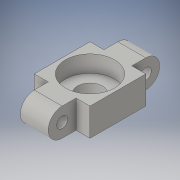
# Autodesk Inventor part: top_anchor_v3
Saved by Autodesk Inventor 2016 (Build 200138000, 138)
## iProperties
Created: 2016-02-24
Part Number: top_anchor_v3
Material: Generic
Document SubType Name: Modeling
Designer: Matt Ruffner
Density: 1 g/cm^3
Appearance: Default
Author: Matt Ruffner
Autodesk Inventor part; units mm, degrees
ref_plane "YZ Plane" through (0, 0, 0) normal (1, 0, 0) x (0, 1, 0)
ref_plane "XZ Plane" through (0, 0, 0) normal (0, 1, 0) x (-1, 0, 0)
ref_plane "XY Plane" through (0, 0, 0) normal (0, 0, 1) x (1, 0, 0)
sketch "Sketch1" plane through (0, 0, 0) normal (0, 1, 0) x (-1, 0, 0)
  line L0 (7.6182, 15.9234) -> (-17.7818, 15.9234)
  line L1 (-17.7818, 15.9234) -> (-17.7818, -34.8766)
  line L2 (-17.7818, -34.8766) -> (7.6182, -34.8766)
  line L3 (7.6182, -34.8766) -> (7.6182, 15.9234)
  line L4 (7.6182, 15.9234) -> (1.2682, 15.9234)
  line L5 (1.2682, 15.9234) -> (1.2682, 3.2234)
  line L6 (1.2682, 3.2234) -> (7.6182, 3.2234)
  line L7 (7.6182, 3.2234) -> (7.6182, 15.9234)
  line L8 (-17.7818, 15.9234) -> (-11.4318, 15.9234)
  line L9 (-11.4318, 15.9234) -> (-11.4318, 3.2234)
  line L10 (-11.4318, 3.2234) -> (-17.7818, 3.2234)
  line L11 (-17.7818, 3.2234) -> (-17.7818, 15.9234)
  line L12 (-17.7818, -34.8766) -> (-11.4318, -34.8766)
  line L13 (-11.4318, -34.8766) -> (-11.4318, -22.1766)
  line L14 (-11.4318, -22.1766) -> (-17.7818, -22.1766)
  line L15 (-17.7818, -22.1766) -> (-17.7818, -34.8766)
  line L16 (7.6182, -34.8766) -> (1.2682, -34.8766)
  line L17 (1.2682, -34.8766) -> (1.2682, -22.1766)
  line L18 (1.2682, -22.1766) -> (7.6182, -22.1766)
  line L19 (7.6182, -22.1766) -> (7.6182, -34.8766)
  circle A0 centre (-5.0818, -9.4766) radius 5.715
  point P0 (0, 0)
  dimension "d0" = 25.4
  dimension "d1" = 50.8
  dimension "d2" = 6.35
  dimension "d3" = 12.7
  dimension "d4" = 6.35
  dimension "d5" = 12.7
  dimension "d6" = 6.35
  dimension "d7" = 12.7
  dimension "d8" = 11.43
  constraints: 40 end point, 10 parallel, 5 horizontal, 5 perpendicular, 2 point on line, 1 centre point
  measures "d0" distance of L2.end L1.end
  measures "d1" distance of L1.end L0.end
  measures "d2" distance of L6.end L5.end
  measures "d3" distance of L5.end L4.end
  measures "d4" distance of L9.end L10.end
  measures "d5" distance of L13.end L12.end
  measures "d6" distance of L17.end L18.end
  measures "d7" distance of L16.end L17.end
  measures "d8" diameter of A0
extrude "Extrusion1" add sketch "Sketch1" along normal blind 12.7 contours L5 L6 L3 L18 L17 L2 L13 L14 L1 L10 L9 L0
sketch "Sketch2" plane through (11.4318, 0, 3.2234) normal (1, 0, 0) x (0, 0, -1)
  line L0 (-12.7, 0) -> (-12.7, 12.7) projected
  line L1 (-12.7, 12.7) -> (0, 12.7) projected
  line L2 (38.1, 12.7) -> (38.1, 0) projected
  circle A0 centre (-6.35, 6.35) radius 2.5083
  circle A1 centre (31.75, 6.35) radius 2.5082
  point P0 (3.2234, 0)
  dimension "d11" = 6.35
  dimension "d12" = 6.35
  dimension "d13" = 6.35
  dimension "d14" = 5.0165
  dimension "d15" = 5.0165
  constraints: 2 centre point, 2 coincident
  measures "d11" distance from line of L0 point (-6.35, 6.35)
  measures "d12" distance from line of point (-6.35, 6.35) L1
  measures "d13" distance from line of L2 point (31.75, 6.35)
  measures "d14" diameter of A0
  measures "d15" diameter of A1
extrude "Extrusion2" cut sketch "Sketch2" against normal through all
sketch "Sketch3" plane through (0, 12.7, 0) normal (0, 1, 0) x (1, 0, 0)
  circle A0 centre (5.0818, 9.4766) radius 5.715 projected
  circle A1 centre (5.0818, 9.4766) radius 11.176
  point P0 (0, 0)
  dimension "d18" = 22.352
  constraints: 1 centre point, 1 coincident
  measures "d18" diameter of A1
extrude "Extrusion3" cut sketch "Sketch3" against normal blind 7.62
fillet "Fillet1" radius 6.35 4 edges at (5.0818, 12.7, 15.9234) (5.0818, 0, 15.9234) (5.0818, 0, -34.8766) (5.0818, 12.7, -34.8766)
body "Solid1"
